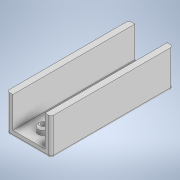
# Autodesk Inventor part: CBCaseMount
Saved by Autodesk Inventor 2020 (Build 240168000, 168)
## iProperties
Created: 2021-05-10
Part Number: CBCaseMount
Material: Generic
Document SubType Name: Modeling
Designer: PAB
Density: 1 g/cm^3
Appearance: Default
Author: PAB
Autodesk Inventor part; units mm, degrees
ref_plane "YZ Plane" through (0, 0, 0) normal (1, 0, 0) x (0, 1, 0)
ref_plane "XZ Plane" through (0, 0, 0) normal (0, 1, 0) x (-1, 0, 0)
ref_plane "XY Plane" through (0, 0, 0) normal (0, 0, 1) x (1, 0, 0)
sketch "Sketch1" plane through (0, 0, 0) normal (0, 1, 0) x (-1, 0, 0)
  line L0 (18.2, 50) -> (-18.2, 50)
  line L1 (-18.2, 50) -> (-18.2, -50)
  line L2 (-18.2, -50) -> (18.2, -50)
  line L3 (18.2, -50) -> (18.2, 50)
  point P0 (0, 0)
  dimension "d0" = 36.4
  dimension "d1" = 100
  constraints: 8 end point, 2 parallel, 1 horizontal, 1 perpendicular
  measures "d0" distance of L2.end L1.end
  measures "d1" distance of L1.end L0.end
extrude "Extrusion1" add sketch "Sketch1" along normal blind 5
sketch "Sketch2" plane through (0, 5, 0) normal (0, 1, 0) x (1, 0, 0)
  circle A0 centre (0, 12.7) radius 4.325
  circle A1 centre (0, -12.7) radius 4.325
  circle A2 centre (0, -38.1) radius 4.325
  circle A3 centre (0, 38.1) radius 4.325
  point P0 (0, 0)
  dimension "d4" = 8.65
  dimension "d5" = 8.65
  dimension "d6" = 8.65
  dimension "d7" = 8.65
  constraints: 4 centre point
  measures "d4" diameter of A0
  measures "d5" diameter of A1
  measures "d6" diameter of A2
  measures "d7" diameter of A3
extrude "Extrusion2" add sketch "Sketch2" along normal blind 5
chamfer "Chamfer1" distance 1.5 angle 45 4 edges at (-4.325, 10, 38.1) (-4.325, 10, 12.7) (-4.325, 10, -12.7) (-4.325, 10, -38.1)
sketch "Sketch3" plane through (0, 5, 0) normal (0, 1, 0) x (1, 0, 0)
  line L0 (-18.2, 50) -> (-18.2, -50) projected
  line L1 (-18.2, -50) -> (18.2, -50) projected
  line L2 (-18.2, 50) -> (-13.2, 50)
  line L3 (-13.2, 50) -> (-13.2, -50)
  line L4 (-13.2, -50) -> (-18.2, -50)
  line L5 (-18.2, -50) -> (-18.2, 50)
  line L6 (18.2, -50) -> (18.2, 50) projected
  line L7 (18.2, 50) -> (13.2, 50)
  line L8 (13.2, 50) -> (13.2, -50)
  line L9 (13.2, -50) -> (18.2, -50)
  line L10 (18.2, -50) -> (18.2, 50)
  point P0 (0, 0)
  dimension "d13" = 5
  dimension "d14" = 5
  constraints: 16 end point, 4 parallel, 2 horizontal, 2 perpendicular, 2 point on line
  measures "d13" distance of L3.end L4.end
  measures "d14" distance of L9.end L8.end
extrude "Extrusion3" add sketch "Sketch3" along normal blind 25.4
sketch "Sketch4" plane through (0, 10, 38.1) normal (0, 1, 0) x (1, 0, 0)
  circle A0 centre (0, 0) radius 2.825 projected
  circle A1 centre (0, 0) radius 2
  circle A2 centre (0, 25.4) radius 2.825 projected
  circle A3 centre (0, 25.4) radius 2
  circle A4 centre (0, 50.8) radius 2.825 projected
  circle A5 centre (0, 50.8) radius 2
  circle A6 centre (0, 76.2) radius 2.825 projected
  circle A7 centre (0, 76.2) radius 2
  point P0 (0, 38.1)
  dimension "d17" = 4
  dimension "d18" = 4
  dimension "d19" = 4
  dimension "d20" = 4
  constraints: 4 centre point, 4 coincident
  measures "d17" diameter of A1
  measures "d18" diameter of A3
  measures "d19" diameter of A5
  measures "d20" diameter of A7
extrude "Extrusion4" cut sketch "Sketch4" against normal blind 25.4 contours A1 | A3 | A5 | A7
sketch "Sketch5" plane through (0, 0, 0) normal (0, -1, 0) x (1, 0, 0)
  circle A0 centre (0, 38.1) radius 2.825 projected
  circle A1 centre (0, 38.1) radius 3
  circle A2 centre (0, 12.7) radius 2 projected
  circle A3 centre (0, 12.7) radius 3
  circle A4 centre (0, -12.7) radius 3
  circle A5 centre (0, -38.1) radius 2 projected
  circle A6 centre (0, -38.1) radius 3
  point P0 (0, 0)
  dimension "d23" = 6
  dimension "d24" = 6
  dimension "d25" = 6
  dimension "d26" = 6
  constraints: 4 centre point, 3 coincident
  measures "d23" diameter of A1
  measures "d24" diameter of A3
  measures "d25" diameter of A4
  measures "d26" diameter of A6
extrude "Extrusion5" cut sketch "Sketch5" against normal blind 2.5 contours A0 | A1 | A2 | A3 | A4 | A5 | A6
fillet "Fillet1" radius 2 8 edges at (-18.2, 0, 0) (0, 0, 50) (18.2, 0, 0) (0, 0, -50) (-18.2, 15.2, -50) (-18.2, 15.2, 50) (18.2, 15.2, 50) (18.2, 15.2, -50)
body "Solid1"
